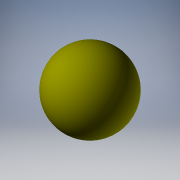
# Autodesk Inventor part: SKF_W 61705-2RS1_PART3
Saved by Autodesk Inventor 2019 (Build 230136000, 136)
## iProperties
Created: 2022-08-30
Part Number: SKF_W 61705-2RS1_PART3
Material: Generic
Catalog Web Link: www.cadenas.de
Description: -Deep groove ball bearings
Vendor: SKF
Document SubType Name: Modeling
Designer: psAdmin
Manufacturer: SKF
Mass: 7 g
Surface Area: 0.0792229 cm^2
Volume: 0.00209677 cm^3
Density: 1 g/cm^3
Appearance: PSOLRGB-192-192-192
Category: PARTsolutions
Company: SKF
Title: SKF_W 61705-2RS1_PART3
Author: Cadenas PARTsolutions
Comments: Deep groove ball bearings
PSOL_IDENT_0: {$CADENAS_DATA/23d-libs/skf/bearings_units_and_housings/ball_bearings/deep_groove_ball_bearings/bb1_
PSOL_IDENT_1: 001_101.prj},211 {VTYP=3D},{NB=SKF_W 61705-2RS1_PART3},{LINA=SKF_W 61705-2RS1_PART3},{NN=BB1_001_101
PSOL_IDENT_2: _PART3},{NOPRJ=TRUE},{DATE=04.08.2022 15:25:15},{GEOMDATE=04.07.2022 10:54:51},{VERSION=},{LINEID=17
PSOL_IDENT_3: 460},{WBVAR=},{WBNUMERIC=}  {NB=SKF_W 61705-2RS1_PART3},{LINA=SKF_W 61705-2RS1_PART3},{KT=DUMMY},{DE
PSOL_IDENT_4: SIGNATION=W 61705-2RS1},{R12=0.20},{DD=25.000},{D=32.000},{B=4.000},{C=},{CX=},{CXX=},{CA=0.000},{XX
PSOL_IDENT_5: VARIANT=},{XXDESIGN=Single row stainless steel},{XXSEALING=Contact seal on both sides},{DESIGN=dgbbw
PSOL_IDENT_6: 2rs},{DESIGNIR=dgbbw2rs},{VARIANT=},{DD1=27.35},{DD2=27.35},{DD2X=},{DD2A=27.35},{D1=29.65},{D1X=0.0
PSOL_IDENT_7: 0},{D2=30.29},{D2A=30.29},{D3=},{D3X=},{D3A=0.000},{D4=},{HH=0.000},{BB=0.000},{BBX=},{BBA=0.000},{F
PSOL_IDENT_8: F=},{R0MAX=0.000},{R0=0.000},{PITCH=28.50},{DW=1.588},{DDAMIN=26.500},{DDAMAX=27.000},{DDBMIN=0.000}
PSOL_IDENT_9: ,{DDBMAX=0.000},{DBMIN=0.000},{DAMAX=31.000},{BBAMIN=0.000},{CAMAX=0.000},{RAMAX=0.200},{LOAD1=0.618
PSOL_IDENT_10: },{LOAD2=0.465},{LOAD3=0.020},{SPEED1=0},{SPEED2=12000},{KR=0.015},{F0=8.800},{Z=21},{II=1},{MASS=0.
PSOL_IDENT_11: 007},{BEARING=W 61705-2RS1},{RING=},{HELP=1.175},{HELP2=0.855},{DD1ALG=13.675},{YALG=13.675},{PITCH1=
PSOL_IDENT_12: 28.500},{DW1=1.588},{YALG1=14.825},{HALG1=1.175},{SH=13.675},{CU=0.482},{HALG=1.175},{B1=0},{SHIELDH
PSOL_IDENT_13: ELP=2},{D4A=0.000},{FFA=0.000},{RS1=},{HELP3=0}
NB: SKF_W 61705-2RS1_PART3
NT: Deep groove ball bearings
NBSYN: SKF_$DESIGNATION._PART3
LINA: SKF_W 61705-2RS1_PART3
CATALOG: SKF
DESIGNATION: W 61705-2RS1
R12: 0.2
DD: 25
D: 32
B: 4
XXDESIGN: Single row stainless steel
XXSEALING: Contact seal on both sides
DD2: 27.35
D2: 30.29
LOAD1: 0.618
LOAD2: 0.465
LOAD3: 0.02
SPEED1: 0
SPEED2: 12000
BEARING: W 61705-2RS1
SUPPLIER: SKF
ARTICLENO: SKF_W 61705-2RS1_PART3
BOMINFO: SKF_W 61705-2RS1_PART3
CREATOR: CADENAS GmbH
Autodesk Inventor part; units mm, degrees
ref_plane "YZ Plane" through (0, 0, 0) normal (1, 0, 0) x (0, 1, 0)
ref_plane "XZ Plane" through (0, 0, 0) normal (0, 1, 0) x (-1, 0, 0)
ref_plane "XY Plane" through (0, 0, 0) normal (0, 0, 1) x (1, 0, 0)
sketch "Sketch_6" plane through (0, 0, 0) normal (0, 0, 1) x (1, 0, 0)
  line L0 (2.794, 14.25) -> (1.206, 14.25)
  arc A0 (2.794, 14.25) -> (1.206, 14.25) centre (2, 14.25) ccw
  line L1 (2.794, 14.25) -> (1.206, 14.25)
  dimension "d0" = 360
  constraints: 4 end point, 2 point on circle, 1 centre point
revolve "Revolution1" add sketch "Sketch_6" angle 360 about axis through (2.794, 14.25, 0) along (1, 0, 0)
body "Solid1"
